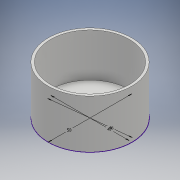
# Autodesk Inventor part: Fill
Saved by Autodesk Inventor 2018 (Build 220112000, 112)
## iProperties
Created: 2019-03-05
Part Number: Fill
Material: Типовые
Document SubType Name: Modeling
Designer: cosko
Density: 1 g/cm^3
Appearance: По умолчанию
Mass: 23.4973 g
Surface Area: 162.756 cm^2
Volume: 23.4973 cm^3
Author: cosko
Autodesk Inventor part; units mm, degrees
ref_plane "YZ Plane" through (0, 0, 0) normal (1, 0, 0) x (0, 1, 0)
ref_plane "XZ Plane" through (0, 0, 0) normal (0, 1, 0) x (-1, 0, 0)
ref_plane "XY Plane" through (0, 0, 0) normal (0, 0, 1) x (1, 0, 0)
sketch "Эскиз1" plane through (0, 0, 0) normal (0, 0, 1) x (1, 0, 0)
  circle A0 centre (0, 0) radius 23 construction
  circle A1 centre (0, 0) radius 23.5
  circle A2 centre (0, 0) radius 25
  dimension "d0" = 46
  dimension "d1" = 47
  dimension "d2" = 50
  constraints: 3 centre point, 3 coincident
  measures "d0" diameter of A0
  measures "d1" diameter of A1
  measures "d2" diameter of A2
extrude "Выдавливание1" add sketch "Эскиз1" along normal blind 3 contours A1 | A2
extrude "Выдавливание2" add sketch "Эскиз1" along normal blind 29
sketch "Эскиз2" plane through (0, 0, 0) normal (0, 0, -1) x (-1, 0, 0)
  arc A0 (0.95, 1.0954) -> (0.95, -1.0954) centre (0, 0) ccw
  line L0 (-1.45, 0) -> (0.95, 0)
  line L1 (0.95, 0) -> (0.95, 1.0954)
  line L2 (0.95, -1.0954) -> (0.95, 1.0954)
  dimension "d7" = 2.9
  dimension "d8" = 2.4
  constraints: 6 end point, 3 point on circle, 1 centre point, 1 coincident, 1 collinear, 1 horizontal, 1 perpendicular, 1 point on line
  measures "d7" diameter of A0
  measures "d8" distance of L0.start L0.end
extrude "Выдавливание3" cut sketch "Эскиз2" against normal blind 10
